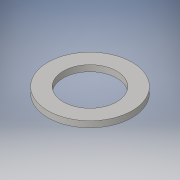
# Autodesk Inventor part: m3_shim
Saved by Autodesk Inventor 2016 (Build 200138000, 138)
## iProperties
Created: 2016-08-18
Part Number: m3_shim
Material: Generic
Document SubType Name: Modeling
Designer: brent
Density: 1 g/cm^3
Appearance: Default
Author: brent
Autodesk Inventor part; units mm, degrees
ref_plane "YZ Plane" through (0, 0, 0) normal (1, 0, 0) x (0, 1, 0)
ref_plane "XZ Plane" through (0, 0, 0) normal (0, 1, 0) x (-1, 0, 0)
ref_plane "XY Plane" through (0, 0, 0) normal (0, 0, 1) x (1, 0, 0)
sketch "Sketch1" plane through (0, 0, 0) normal (0, 1, 0) x (-1, 0, 0)
  circle A0 centre (0, 0) radius 1.75
  circle A1 centre (0, 0) radius 2.75
  dimension "d0" = 3.5
  dimension "d4" = 1
  constraints: 2 centre point, 2 coincident
  measures "d0" diameter of A0
  measures "d4" radial gap between concentric circles of A1 A0
extrude "Extrusion1" add sketch "Sketch1" along normal blind 0.4
body "Solid1"
